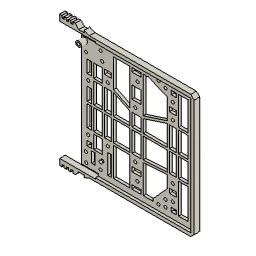
Rack and Dock v2 v74 (Autodesk Fusion 360 design; units mm, degrees)
Autodesk Fusion 360 part; units mm, degrees
(part 1 of 4)
sketch "Base Shape" plane through (0, 0, 0) normal (0, 1, 0) x (1, 0, 0) in component "Card Plate"
  line L0 (0, 0) -> (0, -50)
  line L1 (0, -50) -> (15, -50)
  line L2 (15, -50) -> (15, -53)
  line L3 (15, -53) -> (-13, -53)
  line L4 (-13, -53) -> (-13, -56.5)
  line L5 (0, 0) -> (103, 0) construction
  line L6 (103, 0) -> (103, -55)
  line L7 (103, -55) -> (15, -55)
  line L8 (15, -55) -> (9.5, -55)
  line L9 (9.5, -55) -> (5, -57)
  line L10 (5, -57) -> (5, -55)
  line L11 (15, -53) -> (15, -55) construction
  line L12 (9.5, -55) -> (5, -55) construction
  line L13 (0, -50) -> (0, -55) construction
  line L14 (5, -55) -> (0, -55)
  line L15 (-13, -56.5) -> (-3, -56.5)
  line L16 (-3, -56.5) -> (0, -55)
  line L17 (15, -52) -> (100, -52)
  line L18 (100, -52) -> (100, 0)
  line L19 (67.9969, -52) -> (67.9969, -55) construction
  line L20 (100, -22.1513) -> (103, -22.1513) construction
  line L21 (0, 0) -> (0, 50)
  line L22 (0, 50) -> (15, 50)
  line L23 (15, 50) -> (15, 53)
  line L24 (15, 53) -> (-13, 53)
  line L25 (-13, 53) -> (-13, 56.5)
  line L26 (-13, 56.5) -> (-3, 56.5)
  line L27 (-3, 56.5) -> (0, 55)
  line L28 (5, 55) -> (0, 55)
  line L29 (5, 57) -> (5, 55)
  line L30 (9.5, 55) -> (5, 57)
  line L31 (15, 55) -> (9.5, 55)
  line L32 (103, 55) -> (15, 55)
  line L33 (15, 52) -> (100, 52)
  line L34 (100, 52) -> (100, 0)
  line L35 (103, 0) -> (103, 55)
  dimension "d1" = 50
  dimension "d2" = 15
  dimension "d3" = 3
  dimension "d4" = 28
  dimension "d5" = 3.5
  dimension "d6" = 103
  dimension "d7" = 55
  dimension "d8" = 5.5
  dimension "d9" = 10
  dimension "d10" = 2
  dimension "d12" = 10
  dimension "d13" = 3
  constraint coincident L0.start L5.start
  constraint vertical L0
  constraint perpendicular L0 L1
  constraint perpendicular L1 L2
  constraint perpendicular L2 L3
  constraint perpendicular L3 L4
  constraint perpendicular L0 L5
  constraint perpendicular L5 L6
  constraint perpendicular L2 L7
  constraint parallel L7 L8
  constraint perpendicular L8 L10
  constraint vertical L11
  constraint horizontal L12
  constraint vertical L13
  constraint perpendicular L13 L14
  constraint perpendicular L4 L15
  constraint coincident L2 L17.start
  constraint perpendicular L2 L17
  constraint coincident L5 L18.end
  constraint perpendicular L5 L18
  constraint coincident L17 L19.start
  constraint coincident L7 L19.end
  constraint perpendicular L7 L19
  constraint coincident L18 L20.start
  constraint coincident L6 L20.end
  constraint perpendicular L6 L20
  constraint equal L19 L20
  constraint symmetric L0.start L5 L21.start
  constraint symmetric L0.end L5 L21.end
  constraint symmetric L1.end L5 L22.end
  constraint symmetric L2.end L5 L23.end
  constraint symmetric L3.end L5 L24.end
  constraint symmetric L4.end L5 L25.end
  constraint symmetric L6.start L5 L35.start
  constraint symmetric L5 L6.end L32.start
  constraint symmetric L5 L7.end L31.start
  constraint symmetric L5 L8.end L30.start
  constraint symmetric L5 L9.end L29.start
  constraint symmetric L5 L10.end L28.start
  constraint symmetric L5 L13.end L27.end
  constraint symmetric L5 L15.end L26.end
  constraint symmetric L5 L17.start L33.start
  constraint symmetric L5 L17.end L33.end
  constraint symmetric L5 L18.end L34.end
  measures "d1" distance of L0.start L0.end
  measures "d2" distance of L0.end L1.end
  measures "d3" distance of L1.end L2.end
  measures "d4" distance of L2.end L3.end
  measures "d5" distance of L3.end L4.end
  measures "d6" distance of L0.start L5.end
  measures "d7" distance of L5.end L6.end
  measures "d8" distance of L7.end L8.end
  measures "d9" horizontal distance of L7.end L9.end
  measures "d10" distance of L9.end L10.end
  measures "d12" distance of L4.end L15.end
  measures "d13" distance of L7 L17
extrude "Extrude1" add sketch "Base Shape" along normal blind 2 makes body 1 in component "Card Plate"
extrude "Extrude2" add sketch "Base Shape" against normal blind 3 contours L2 L3 L4 L6 L7 L8 L9 L10 L14 L15 L16 L17 L18 L23 L24 L25 L26 L27 L28 L29 L30 L31 L32 L33 L34 L35 bodies 1 in component "Card Plate"
chamfer "Chamfer1" distance 3 angle 45 2 edges at (103, -0.5, 55) (103, -0.5, -55) on bodies 1 in component "Card Plate"
sketch "Knurling" plane through (0, -3, 0) normal (0, -1, 0) x (1, 0, 0) in component "Card Plate"
  line L0 (100, -55) -> (103, -52)
  line L1 (103, -52) -> (103, 52)
  line L2 (103, 52) -> (100, 55)
  line L3 (100, 55) -> (9.5, 55)
  line L4 (9.5, 55) -> (5, 57)
  line L5 (5, 57) -> (5, 55)
  line L6 (5, 55) -> (0, 55)
  line L7 (0, 55) -> (-3, 56.5)
  line L8 (-3, 56.5) -> (-13, 56.5)
  line L9 (-13, 56.5) -> (-13, 53)
  line L10 (-13, 53) -> (15, 53)
  line L11 (15, 53) -> (15, 52)
  line L12 (15, 52) -> (100, 52)
  line L13 (100, 52) -> (100, -52)
  line L14 (100, -52) -> (15, -52)
  line L15 (15, -52) -> (15, -53)
  line L16 (15, -53) -> (-13, -53)
  line L17 (-13, -53) -> (-13, -56.5)
  line L18 (-13, -56.5) -> (-3, -56.5)
  line L19 (-3, -56.5) -> (0, -55)
  line L20 (0, -55) -> (5, -55)
  line L21 (5, -55) -> (5, -57)
  line L22 (5, -57) -> (9.5, -55)
  line L23 (9.5, -55) -> (100, -55)
  line L24 (-12, 56.5) -> (-12, 55.5)
  line L25 (-12, 55.5) -> (-11, 55.5)
  line L26 (-11, 55.5) -> (-11, 56.5)
  line L27 (0, 0) -> (100, 0) construction
  line L28 (-12, -56.5) -> (-12, -55.5)
  line L29 (-12, -55.5) -> (-11, -55.5)
  line L30 (-11, -55.5) -> (-11, -56.5)
  line L31 (-10.125, 56.5) -> (-10.125, 55.5)
  line L32 (-10.125, 55.5) -> (-9.125, 55.5)
  line L33 (-9.125, 55.5) -> (-9.125, 56.5)
  line L34 (-10.125, -56.5) -> (-10.125, -55.5)
  line L35 (-10.125, -55.5) -> (-9.125, -55.5)
  line L36 (-9.125, -55.5) -> (-9.125, -56.5)
  line L37 (-8.25, 56.5) -> (-8.25, 55.5)
  line L38 (-8.25, 55.5) -> (-7.25, 55.5)
  line L39 (-7.25, 55.5) -> (-7.25, 56.5)
  line L40 (-8.25, -56.5) -> (-8.25, -55.5)
  line L41 (-8.25, -55.5) -> (-7.25, -55.5)
  line L42 (-7.25, -55.5) -> (-7.25, -56.5)
  line L43 (-6.375, 56.5) -> (-6.375, 55.5)
  line L44 (-6.375, 55.5) -> (-5.375, 55.5)
  line L45 (-5.375, 55.5) -> (-5.375, 56.5)
  line L46 (-6.375, -56.5) -> (-6.375, -55.5)
  line L47 (-6.375, -55.5) -> (-5.375, -55.5)
  line L48 (-5.375, -55.5) -> (-5.375, -56.5)
  line L49 (-4.5, 56.5) -> (-4.5, 55.5)
  line L50 (-4.5, 55.5) -> (-3.5, 55.5)
  line L51 (-3.5, 55.5) -> (-3.5, 56.5)
  line L52 (-4.5, -56.5) -> (-4.5, -55.5)
  line L53 (-4.5, -55.5) -> (-3.5, -55.5)
  line L54 (-3.5, -55.5) -> (-3.5, -56.5)
  dimension "d19" = 1
  dimension "d20" = 1
  dimension "d21" = 1
  dimension "d24" = 7.5
  dimension "d25" = 0
  constraint coincident L8 L24.start
  constraint perpendicular L8 L24
  constraint perpendicular L24 L25
  constraint coincident L8 L26.end
  constraint perpendicular L8 L26
  constraint coincident L27.start origin
  constraint midpoint L13 L27.end
  constraint symmetric L24.start L27 L28.start
  constraint symmetric L24.end L27 L28.end
  constraint symmetric L25.end L27 L29.end
  constraint symmetric L26.end L27 L30.end
  measures "d19" distance of L24.start L24.end
  measures "d20" distance of L24.end L25.end
  measures "d21" distance of L8.end L24.start
extrude "Extrude6" cut sketch "Knurling" against normal blind 20 contours L18 L52 L53 L54 | L18 L46 L47 L48 | L8 L49 L50 L51 | L18 L40 L41 L42 | L8 L43 L44 L45 | L18 L34 L35 L36 | L8 L37 L38 L39 | L18 L28 L29 L30 | L8 L31 L32 L33 | L8 L24 L25 L26 bodies 1 in component "Card Plate"
sketch "Base Shape (2)" plane through (0, 2, 0) normal (0, 1, 0) x (-1, 0, 0) in component "Bay Body"
  line L0 (-15, -53) -> (-15, -50)
  line L1 (-15, -50) -> (0, -50)
  line L2 (0, -50) -> (0, 50)
  line L3 (0, 50) -> (-15, 50)
  line L4 (-15, 50) -> (-15, 53)
  line L5 (-5, 55) -> (0, 55)
  line L6 (-5, 57) -> (-5, 55)
  line L7 (-9.5, 55) -> (-5, 57)
  line L8 (-100, 55) -> (-9.5, 55)
  line L9 (-100, 55) -> (-103, 52)
  line L10 (-103, 52) -> (-103, 0) construction
  line L11 (-103.2, 52.0828) -> (-103.2, 0)
  line L12 (-100.0828, 55.2) -> (-103.2, 52.0828)
  line L13 (-100.0828, 55.2) -> (-9.5424, 55.2)
  line L14 (-9.5424, 55.2) -> (-4.8, 57.3078)
  line L15 (-4.8, 57.3078) -> (-4.8, 55.2)
  line L16 (-4.8, 55.2) -> (0, 55.2)
  line L17 (-103, 0) -> (0, 0) construction
  circle A0 centre (-14, 60.2) radius 2.25
  line L18 (-51.5, 0) -> (-51.5, 68.1067) construction
  circle A1 centre (-96.5, 60.2) radius 2.25
  line L19 (-96.5, 60.2) -> (-51.5, 60.2) construction
  line L20 (-14, 60.2) -> (-51.5, 60.2) construction
  line L21 (-96.5, 60.2) -> (-96.5, 55.2) construction
  line L22 (-14, 60.2) -> (-14, 55.2) construction
  line L23 (0, 55.2) -> (0, 65.2) construction
  line L24 (-108.2, 60.2) -> (-108.2, 0)
  line L25 (0, 60.2) -> (-7.3, 60.2)
  line L26 (-7.3, 60.2) -> (-7.3, 65.2)
  line L27 (-7.3, 65.2) -> (-20.7, 65.2)
  line L28 (-14, 60.2) -> (-14, 65.2) construction
  line L29 (-20.7, 60.2) -> (-51.5, 60.2)
  line L30 (-20.7, 65.2) -> (-20.7, 60.2)
  line L31 (0, 60.2) -> (0, 55.2)
  line L32 (-96.5, 60.2) -> (-96.5, 65.2) construction
  line L33 (-89.8, 65.2) -> (-103.2, 65.2)
  line L34 (-89.8, 65.2) -> (-89.8, 60.2)
  line L35 (-103.2, 65.2) -> (-103.2, 60.2)
  line L36 (-89.8, 60.2) -> (-51.5, 60.2)
  line L37 (-103.2, 60.2) -> (-108.2, 60.2)
  line L38 (-4.8, -55.2) -> (0, -55.2)
  line L39 (-4.8, -57.3078) -> (-4.8, -55.2)
  line L40 (-9.5424, -55.2) -> (-4.8, -57.3078)
  line L41 (-100.0828, -55.2) -> (-9.5424, -55.2)
  line L42 (-100.0828, -55.2) -> (-103.2, -52.0828)
  line L43 (-103.2, -52.0828) -> (-103.2, 0)
  line L44 (0, -60.2) -> (0, -55.2)
  line L45 (0, -60.2) -> (-7.3, -60.2)
  line L46 (-7.3, -60.2) -> (-7.3, -65.2)
  line L47 (-7.3, -65.2) -> (-20.7, -65.2)
  line L48 (-20.7, -65.2) -> (-20.7, -60.2)
  circle A2 centre (-14, -60.2) radius 2.25
  line L49 (-20.7, -60.2) -> (-51.5, -60.2)
  line L50 (-89.8, -60.2) -> (-51.5, -60.2)
  line L51 (-89.8, -65.2) -> (-89.8, -60.2)
  line L52 (-89.8, -65.2) -> (-103.2, -65.2)
  line L53 (-103.2, -65.2) -> (-103.2, -60.2)
  line L54 (-103.2, -60.2) -> (-108.2, -60.2)
  line L55 (-108.2, -60.2) -> (-108.2, 0)
  circle A3 centre (-96.5, -60.2) radius 2.25
  line L56 (-67.2166, 55.2) -> (-67.2166, 60.2) construction
  line L57 (-103.2, 0) -> (-108.2, 0) construction
  line L58 (8.25, -55.5) -> (8.25, -56.5)
  line L59 (8.25, -56.5) -> (9.125, -56.5)
  line L60 (9.125, -56.5) -> (9.125, -55.5)
  line L61 (9.125, -55.5) -> (10.125, -55.5)
  line L62 (10.125, -55.5) -> (10.125, -56.5)
  line L63 (10.125, -56.5) -> (11, -56.5)
  line L64 (11, -56.5) -> (11, -55.5)
  line L65 (11, -55.5) -> (12, -55.5)
  line L66 (12, -55.5) -> (12, -56.5)
  line L67 (12, -56.5) -> (13, -56.5)
  line L68 (13, -56.5) -> (13, -53)
  line L69 (13, -53) -> (-15, -53)
  line L70 (-15, 53) -> (13, 53)
  line L71 (13, 53) -> (13, 56.5)
  line L72 (13, 56.5) -> (12, 56.5)
  line L73 (12, 56.5) -> (12, 55.5)
  line L74 (12, 55.5) -> (11, 55.5)
  line L75 (11, 55.5) -> (11, 56.5)
  line L76 (11, 56.5) -> (10.125, 56.5)
  line L77 (10.125, 56.5) -> (10.125, 55.5)
  line L78 (10.125, 55.5) -> (9.125, 55.5)
  line L79 (9.125, 55.5) -> (9.125, 56.5)
  line L80 (9.125, 56.5) -> (8.25, 56.5)
  line L81 (8.25, 56.5) -> (8.25, 55.5)
  line L82 (8.25, 55.5) -> (7.25, 55.5)
  line L83 (7.25, 55.5) -> (7.25, 56.5)
  line L84 (7.25, 56.5) -> (6.375, 56.5)
  line L85 (6.375, 56.5) -> (6.375, 55.5)
  line L86 (6.375, 55.5) -> (5.375, 55.5)
  line L87 (5.375, 55.5) -> (5.375, 56.5)
  line L88 (5.375, 56.5) -> (4.5, 56.5)
  line L89 (4.5, 56.5) -> (4.5, 55.5)
  line L90 (4.5, 55.5) -> (3.5, 55.5)
  line L91 (3.5, 55.5) -> (3.5, 56.5)
  line L92 (3.5, 56.5) -> (3, 56.5)
  line L93 (3, 56.5) -> (0, 55)
  line L94 (0, 55) -> (-5, 55)
  line L95 (-5, 55) -> (-5, 57)
  line L96 (-5, 57) -> (-9.5, 55)
  line L97 (-9.5, 55) -> (-100, 55)
  line L98 (-100, 55) -> (-103, 52)
  line L99 (-103, -52) -> (-100, -55)
  line L100 (-100, -55) -> (-9.5, -55)
  line L101 (-9.5, -55) -> (-5, -57)
  line L102 (-5, -57) -> (-5, -55)
  line L103 (-5, -55) -> (0, -55)
  line L104 (0, -55) -> (3, -56.5)
  line L105 (3, -56.5) -> (3.5, -56.5)
  line L106 (3.5, -56.5) -> (3.5, -55.5)
  line L107 (3.5, -55.5) -> (4.5, -55.5)
  line L108 (4.5, -55.5) -> (4.5, -56.5)
  line L109 (4.5, -56.5) -> (5.375, -56.5)
  line L110 (5.375, -56.5) -> (5.375, -55.5)
  line L111 (5.375, -55.5) -> (6.375, -55.5)
  line L112 (6.375, -55.5) -> (6.375, -56.5)
  line L113 (6.375, -56.5) -> (7.25, -56.5)
  line L114 (7.25, -56.5) -> (7.25, -55.5)
  line L115 (7.25, -55.5) -> (8.25, -55.5)
  dimension "d28" = 0.2
  dimension "d29" = 4.5
  dimension "d30" = 4.5
  dimension "d31" = 5
  dimension "d32" = 37.5
  dimension "d33" = 5
  dimension "d35" = 13.4
  dimension "d36" = 45
  constraint coincident L9.end L10.start
  constraint coincident L17.end origin
  constraint perpendicular L2 L17
  constraint midpoint L17 L18.start
  constraint perpendicular L17 L18
  constraint coincident A1.centre L19.start
  constraint coincident L18 L19.end
  constraint perpendicular L18 L19
  constraint coincident A0.centre L20.start
  constraint perpendicular L18 L20
  constraint coincident L13 L21.end
  constraint perpendicular L13 L21
  constraint coincident L13 L22.end
  constraint perpendicular L13 L22
  constraint equal L21 L22
  constraint perpendicular L16 L23
  constraint vertical L10
  constraint perpendicular L17 L24
  constraint coincident L23 L25.start
  constraint perpendicular L23 L25
  constraint midpoint L27 L28.end
  constraint vertical L28
  constraint equal L22 L28
  constraint perpendicular L18 L29
  constraint vertical L26
  constraint perpendicular L27 L30
  constraint vertical L30
  constraint equal L26 L30
  constraint perpendicular L19 L32
  constraint equal L28 L32
  constraint perpendicular L32 L33
  constraint midpoint L32.end L33
  constraint coincident L19 L34.end
  constraint perpendicular L19 L34
  constraint perpendicular L33 L35
  constraint coincident L24 L37.end
  constraint perpendicular L24 L37
  constraint equal L27 L33
  constraint symmetric L11.start L17 L42.end
  constraint symmetric L11.end L17 L43.end
  constraint symmetric L12.start L17 L41.start
  constraint symmetric L13.end L17 L40.start
  constraint symmetric L14.end L17 L39.start
  constraint symmetric L15.end L17 L38.start
  constraint symmetric L16.end L17 L38.end
  constraint symmetric L17 A0 A2
  constraint symmetric L17 A1 A3
  constraint symmetric L17 L24.end L55.end
  constraint symmetric L17 L25.start L44.start
  constraint symmetric L17 L25.end L45.end
  constraint symmetric L17 L26.end L46.end
  constraint symmetric L17 L27.end L47.end
  constraint symmetric L17 L29.start L48.end
  constraint symmetric L17 L19.end L49.end
  constraint symmetric L17 L33.start L51.start
  constraint symmetric L17 L33.end L52.end
  constraint symmetric L17 L34.end L50.start
  constraint symmetric L17 L35.end L53.end
  constraint symmetric L17 L24.start L54.end
  constraint coincident L13 L56.start
  constraint coincident L36 L56.end
  constraint perpendicular L36 L56
  constraint perpendicular L43 L57
  constraint equal L56 L57
  constraint equal L34 L35
  measures "d29" diameter of A0
  measures "d30" diameter of A1
  measures "d31" distance of A0.centre L22.end
  measures "d32" distance of A0.centre L19.end
  measures "d33" vertical distance of L25.end L26.end
  measures "d35" distance of L26.end L27.end
  measures "d36" distance of L18 A1.centre
extrude "Extrude1'" add sketch "Base Shape (2)" against normal blind 5.5 separate body makes body 2 in component "Bay Body"
sketch "Backing Tab" plane through (0, 2, 0) normal (0, 1, 0) x (-1, 0, 0) in component "Bay Body"
  circle A0 centre (-96.5, -60.2) radius 2.25
  circle A1 centre (-96.5, 60.2) radius 2.25
  circle A2 centre (-14, -60.2) radius 2.25
  circle A3 centre (-14, 60.2) radius 2.25
  line L0 (-89.8, -65.2) -> (-89.8, -60.2)
  line L1 (-89.8, -60.2) -> (-20.7, -60.2)
  line L2 (-20.7, -60.2) -> (-20.7, -65.2)
  line L3 (-20.7, -65.2) -> (-7.3, -65.2)
  line L4 (-7.3, -65.2) -> (-7.3, -60.2)
  line L5 (-7.3, -60.2) -> (0, -60.2)
  line L6 (0, -60.2) -> (0, -55.2)
  line L7 (0, -55.2) -> (-4.8, -55.2)
  line L8 (-4.8, -55.2) -> (-4.8, -57.3078)
  line L9 (-4.8, -57.3078) -> (-9.5424, -55.2)
  line L10 (-9.5424, -55.2) -> (-100.0828, -55.2)
  line L11 (-100.0828, -55.2) -> (-103.2, -52.0828)
  line L12 (-103.2, -52.0828) -> (-103.2, 52.0828)
  line L13 (-103.2, 52.0828) -> (-100.0828, 55.2)
  line L14 (-100.0828, 55.2) -> (-9.5424, 55.2)
  line L15 (-9.5424, 55.2) -> (-4.8, 57.3078)
  line L16 (-4.8, 57.3078) -> (-4.8, 55.2)
  line L17 (-4.8, 55.2) -> (0, 55.2)
  line L18 (0, 55.2) -> (0, 60.2)
  line L19 (0, 60.2) -> (-7.3, 60.2)
  line L20 (-7.3, 60.2) -> (-7.3, 65.2)
  line L21 (-7.3, 65.2) -> (-20.7, 65.2)
  line L22 (-20.7, 65.2) -> (-20.7, 60.2)
  line L23 (-20.7, 60.2) -> (-89.8, 60.2)
  line L24 (-89.8, 60.2) -> (-89.8, 65.2)
  line L25 (-89.8, 65.2) -> (-103.2, 65.2)
  line L26 (-103.2, 65.2) -> (-103.2, 60.2)
  line L27 (-103.2, 60.2) -> (-108.2, 60.2)
  line L28 (-108.2, 60.2) -> (-108.2, -60.2)
  line L29 (-108.2, -60.2) -> (-103.2, -60.2)
  line L30 (-103.2, -60.2) -> (-103.2, -65.2)
  line L31 (-103.2, -65.2) -> (-89.8, -65.2)
  line L32 (0, 55.2) -> (0, 52)
  line L33 (0, 52) -> (-100, 52)
  line L34 (0, 0) -> (-118.983, 0) construction
  line L35 (-100, 52) -> (-100, 0)
  line L36 (0, -55.2) -> (0, -52)
  line L37 (0, -52) -> (-100, -52)
  line L38 (-100, -52) -> (-100, 0)
  dimension "d48" = 3.2
  dimension "d49" = 3.2
  constraint coincident L17.end L18.start
  constraint perpendicular L17 L32
  constraint perpendicular L32 L33
  constraint coincident L34.start origin
  constraint perpendicular L28 L34
  constraint coincident L34 L35.end
  constraint perpendicular L34 L35
  constraint symmetric L17.end L34 L6.end
  constraint symmetric L32.end L34 L36.end
  constraint symmetric L33.end L34 L37.end
  constraint symmetric L34 L35.end L38.end
  measures "d48" distance of L17.end L32.end
  measures "d49" distance of L12 L33.end
extrude "Extrude3" add sketch "Backing Tab" along normal blind 2 bodies 2 in component "Bay Body"
chamfer "Chamfer8" distance 2.5 angle 45 8 edges at (7.3, 0.25, 65.2) (20.7, 0.25, 65.2) (89.8, 0.25, 65.2) (103.2, 0.25, 65.2) (103.2, 0.25, -65.2) (89.8, 0.25, -65.2) (20.7, 0.25, -65.2) (7.3, 0.25, -65.2) on bodies 2 in component "Bay Body"
chamfer "Chamfer9" distance 2.5 angle 45 8 edges at (103.2, 0.25, 60.2) (89.8, 0.25, 60.2) (7.3, 0.25, 60.2) (20.7, 0.25, 60.2) (103.2, 0.25, -60.2) (89.8, 0.25, -60.2) (7.3, 0.25, -60.2) (20.7, 0.25, -60.2) on bodies 2 in component "Bay Body"
chamfer "Chamfer10" distance 2.5 angle 45 2 edges at (108.2, 0.25, 60.2) (108.2, 0.25, -60.2) on bodies 2 in component "Bay Body"
chamfer "Chamfer11" distance 1 angle 45 2 edges at (0, 0.25, 60.2) (0, 0.25, -60.2) on bodies 2 in component "Bay Body"
sketch "extra material near tab" plane through (0, -3.5, 0) normal (0, -1, 0) x (1, 0, 0) in component "Bay Body"
  line L0 (0, -59.2) -> (1, -60.2)
  line L1 (1, -60.2) -> (4.8, -60.2)
  line L2 (4.8, -60.2) -> (9.8, -65.2)
  line L3 (9.8, -65.2) -> (18.2, -65.2)
  line L4 (18.2, -65.2) -> (23.2, -60.2)
  line L5 (23.2, -60.2) -> (87.3, -60.2)
  line L6 (87.3, -60.2) -> (92.3, -65.2)
  line L7 (92.3, -65.2) -> (100.7, -65.2)
  line L8 (100.7, -65.2) -> (108.2, -57.7)
  line L9 (108.2, -57.7) -> (108.2, 57.7)
  line L10 (108.2, 57.7) -> (100.7, 65.2)
  line L11 (100.7, 65.2) -> (92.3, 65.2)
  line L12 (92.3, 65.2) -> (87.3, 60.2)
  line L13 (87.3, 60.2) -> (23.2, 60.2)
  line L14 (23.2, 60.2) -> (18.2, 65.2)
  line L15 (18.2, 65.2) -> (9.8, 65.2)
  line L16 (9.8, 65.2) -> (4.8, 60.2)
  line L17 (4.8, 60.2) -> (1, 60.2)
  line L18 (1, 60.2) -> (0, 59.2)
  line L19 (0, 59.2) -> (0, 55.2)
  line L20 (0, 55.2) -> (4.8, 55.2)
  line L21 (4.8, 55.2) -> (4.8, 57.3078)
  line L22 (4.8, 57.3078) -> (9.5424, 55.2)
  line L23 (9.5424, 55.2) -> (100.0828, 55.2)
  line L24 (100.0828, 55.2) -> (103.2, 52.0828)
  line L25 (103.2, 52.0828) -> (103.2, -52.0828)
  line L26 (103.2, -52.0828) -> (100.0828, -55.2)
  line L27 (100.0828, -55.2) -> (9.5424, -55.2)
  line L28 (9.5424, -55.2) -> (4.8, -57.3078)
  line L29 (4.8, -57.3078) -> (4.8, -55.2)
  line L30 (4.8, -55.2) -> (0, -55.2)
  line L31 (0, -55.2) -> (0, -59.2)
  circle A0 centre (96.5, -60.2) radius 2.25
  circle A1 centre (96.5, 60.2) radius 2.25
  circle A2 centre (14, -60.2) radius 2.25
  circle A3 centre (14, 60.2) radius 2.25
  line L32 (0, 59.2) -> (2.1078, 61.3078)
  line L33 (2.1078, 61.3078) -> (5.9078, 61.3078)
  line L34 (0, 0) -> (31.4782, 0) construction
  line L35 (0, -59.2) -> (2.1078, -61.3078)
  line L36 (2.1078, -61.3078) -> (5.9078, -61.3078)
  dimension "d56" = 4
  constraint coincident L18.end L19.start
  constraint parallel L18 L32
  constraint coincident L16 L33.end
  constraint parallel L17 L33
  constraint coincident L34.start origin
  constraint perpendicular L25 L34
  constraint symmetric L18.end L34 L0.start
  constraint symmetric L32.end L34 L35.end
  constraint symmetric L33.end L34 L36.end
  measures "d56" distance of L21.end L33
extrude "Extrude4" add sketch "extra material near tab" against normal blind 7.5 contours L1 L2 L35 L36 | L16 L17 L32 L33 bodies 2 in component "Bay Body"
sketch "Base Shape (3)" plane through (0, 4, 0) normal (0, 1, 0) x (-1, 0, 0) in component "End Frame A"
  circle A0 centre (-14, 60.2) radius 2.25
  circle A1 centre (-14, -60.2) radius 2.25
  circle A2 centre (-96.5, 60.2) radius 2.25
  circle A3 centre (-96.5, -60.2) radius 2.25
  line L0 (-2.1078, -61.3078) -> (0, -59.2)
  line L1 (0, -59.2) -> (0, -52)
  line L2 (0, -52) -> (-100, -52)
  line L3 (-100, -52) -> (-100, 52)
  line L4 (-100, 52) -> (0, 52)
  line L5 (0, 52) -> (0, 59.2)
  line L6 (0, 59.2) -> (-2.1078, 61.3078)
  line L7 (-2.1078, 61.3078) -> (-5.9078, 61.3078)
  line L8 (-5.9078, 61.3078) -> (-9.8, 65.2)
  line L9 (-9.8, 65.2) -> (-18.2, 65.2)
  line L10 (-18.2, 65.2) -> (-23.2, 60.2)
  line L11 (-23.2, 60.2) -> (-87.3, 60.2)
  line L12 (-87.3, 60.2) -> (-92.3, 65.2)
  line L13 (-92.3, 65.2) -> (-100.7, 65.2)
  line L14 (-100.7, 65.2) -> (-108.2, 57.7)
  line L15 (-108.2, 57.7) -> (-108.2, -57.7)
  line L16 (-108.2, -57.7) -> (-100.7, -65.2)
  line L17 (-100.7, -65.2) -> (-92.3, -65.2)
  line L18 (-92.3, -65.2) -> (-87.3, -60.2)
  line L19 (-87.3, -60.2) -> (-23.2, -60.2)
  line L20 (-23.2, -60.2) -> (-18.2, -65.2)
  line L21 (-18.2, -65.2) -> (-9.8, -65.2)
  line L22 (-9.8, -65.2) -> (-5.9078, -61.3078)
  line L23 (-5.9078, -61.3078) -> (-2.1078, -61.3078)
  line L24 (-96.5, 60.2) -> (-14, 60.2) construction
  line L25 (-96.5, -60.2) -> (-14, -60.2) construction
  line L26 (-55.25, -60.2) -> (-55.25, 60.2) construction
  line L27 (-55.25, 0) -> (-108.2, 0) construction
  line L28 (-55.25, 60.2) -> (-87.3, 60.2)
  line L29 (-87.3, 60.2) -> (-92.3, 65.2)
  line L30 (-92.3, 65.2) -> (-100.7, 65.2)
  line L31 (-100.7, 65.2) -> (-108.2, 57.7)
  line L32 (-108.2, 57.7) -> (-108.2, 0)
  circle A4 centre (-96.5, 60.2) radius 2.25
  line L33 (-55.25, 60.2) -> (-23.2, 60.2)
  line L34 (-23.2, 60.2) -> (-18.2, 65.2)
  line L35 (-18.2, 65.2) -> (-9.8, 65.2)
  line L36 (-9.8, 65.2) -> (-2.3, 57.7)
  line L37 (-2.3, 57.7) -> (-2.3, 0)
  circle A5 centre (-14, 60.2) radius 2.25
  line L38 (-108.2, -57.7) -> (-108.2, 0)
  line L39 (-100.7, -65.2) -> (-108.2, -57.7)
  line L40 (-92.3, -65.2) -> (-100.7, -65.2)
  line L41 (-87.3, -60.2) -> (-92.3, -65.2)
  line L42 (-55.25, -60.2) -> (-87.3, -60.2)
  line L43 (-23.2, -60.2) -> (-18.2, -65.2)
  line L44 (-55.25, -60.2) -> (-23.2, -60.2)
  line L45 (-18.2, -65.2) -> (-9.8, -65.2)
  line L46 (-9.8, -65.2) -> (-2.3, -57.7)
  line L47 (-2.3, -57.7) -> (-2.3, 0)
  circle A6 centre (-96.5, -60.2) radius 2.25
  circle A7 centre (-14, -60.2) radius 2.25
  constraint coincident A2.centre L24.start
  constraint coincident A0.centre L24.end
  constraint coincident A3.centre L25.start
  constraint coincident A1.centre L25.end
  constraint midpoint L25 L26.start
  constraint midpoint L24 L26.end
  constraint midpoint L26 L27.start
  constraint midpoint L15 L27.end
  constraint coincident L11.end L12.start
  constraint coincident L12.end L13.start
  constraint coincident L13.end L14.start
  constraint coincident L14.end L15.start
  constraint concentric A2 A4
  constraint symmetric L28.start L26 L33.start
  constraint symmetric L26 L27.end L37.end
  constraint symmetric L26 L11.end L10.end
  constraint symmetric L26 L12.end L9.end
  constraint symmetric L26 L13.end L8.end
  constraint symmetric L26 L14.end L36.end
  constraint symmetric L26 A4 A5
  constraint symmetric L26.end L27 L26.start
  constraint symmetric L32.end L27 L38.end
  constraint symmetric L27 L11.end L18.end
  constraint symmetric L27 L12.end L17.end
  constraint symmetric L27 L13.end L16.end
  constraint symmetric L27 L14.end L15.end
  constraint symmetric L27 A4 A6
  constraint symmetric L27 L26.end L26.start
  constraint symmetric L27 L10.end L19.end
  constraint symmetric L27 L9.end L20.end
  constraint symmetric L27 L8.end L21.end
  constraint symmetric L27 L36.end L46.end
  constraint symmetric L27 L37.end L47.end
  constraint symmetric L27 A5 A7
extrude "Extrude1''" add sketch "Base Shape (3)" along normal blind 3 separate body contours A0 A5 | A1 A7 | A2 A4 | A3 A6 | L2 L3 L4 L8 L9 L10 L11 L12 L13 L14 L15 L16 L17 L18 L19 L20 L21 L22 L28 L29 L30 L31 L32 L33 L34 L35 L36 L37 L38 L39 L40 L41 L42 L43 L44 L45 L46 L47 | L2 L3 L4 L37 L47 makes body 3 in component "End Frame A"
sketch "Bar Holder" plane through (0, 4, 0) normal (0, -1, 0) x (1, 0, 0) in component "End Frame A"
  line L0 (23.2, -60.2) -> (87.3, -60.2)
  line L1 (87.3, -60.2) -> (92.3, -65.2)
  line L2 (92.3, -65.2) -> (100.7, -65.2)
  line L3 (100.7, -65.2) -> (108.2, -57.7)
  line L4 (108.2, -57.7) -> (108.2, 57.7)
  line L5 (108.2, 57.7) -> (100.7, 65.2)
  line L6 (100.7, 65.2) -> (92.3, 65.2)
  line L7 (92.3, 65.2) -> (87.3, 60.2)
  line L8 (87.3, 60.2) -> (23.2, 60.2)
  line L9 (23.2, 60.2) -> (18.2, 65.2)
  line L10 (18.2, 65.2) -> (9.8, 65.2)
  line L11 (9.8, 65.2) -> (2.3, 57.7)
  line L12 (2.3, 57.7) -> (2.3, -57.7)
  line L13 (2.3, -57.7) -> (9.8, -65.2)
  line L14 (9.8, -65.2) -> (18.2, -65.2)
  line L15 (18.2, -65.2) -> (23.2, -60.2)
  circle A0 centre (14, 60.2) radius 2.25
  line L16 (55.25, 60.2) -> (55.25, -60.2) construction
  line L17 (108.2, 0) -> (2.3, 0) construction
  line L18 (11.75, 60.2) -> (16.25, 60.2) construction
  line L19 (16.25, 60.2) -> (16.25, 65.2)
  line L20 (16.25, 65.2) -> (19.7855, 68.7355)
  line L21 (11.75, 65.2) -> (16.75, 65.2) construction
  line L22 (19.7855, 68.7355) -> (22.5433, 68.7355)
  line L23 (22.5433, 68.7355) -> (18.6039, 64.7961)
  line L24 (22.5433, 68.7355) -> (26.8209, 68.7355) construction
  line L25 (18.2, 65.2) -> (18.2, 60.2)
  circle A1 centre (14, 60.2) radius 4.2
  line L26 (18.4731, 67.4231) -> (19.852, 66.0443) construction
  line L27 (18.6039, 64.7961) -> (18.2, 64.3923)
  line L28 (14, 60.2) -> (14, 62.45) construction
  line L29 (5.4567, 68.7355) -> (9.3961, 64.7961)
  line L30 (8.2145, 68.7355) -> (5.4567, 68.7355)
  line L31 (11.75, 65.2) -> (8.2145, 68.7355)
  line L32 (11.75, 60.2) -> (11.75, 65.2)
  line L33 (9.8, 65.2) -> (9.8, 60.2)
  line L34 (9.3961, 64.7961) -> (9.8, 64.3923)
  circle A2 centre (14, 60.2) radius 2.25
  circle A3 centre (96.5, 60.2) radius 2.25
  circle A4 centre (14, -60.2) radius 2.25
  line L35 (98.75, 65.2) -> (102.2855, 68.7355)
  line L36 (102.2855, 68.7355) -> (105.0433, 68.7355)
  line L37 (105.0433, 68.7355) -> (101.1039, 64.7961)
  line L38 (101.1039, 64.7961) -> (100.7, 64.3923)
  line L39 (100.7, 65.2) -> (100.7, 60.2)
  line L40 (98.75, 60.2) -> (98.75, 65.2)
  circle A5 centre (96.5, 60.2) radius 4.2
  circle A6 centre (96.5, 60.2) radius 2.25
  line L41 (94.25, 60.2) -> (94.25, 65.2)
  line L42 (92.3, 65.2) -> (92.3, 60.2)
  line L43 (91.8961, 64.7961) -> (92.3, 64.3923)
  line L44 (87.9567, 68.7355) -> (91.8961, 64.7961)
  line L45 (94.25, 65.2) -> (90.7145, 68.7355)
  line L46 (90.7145, 68.7355) -> (87.9567, 68.7355)
  line L47 (16.25, -55.2) -> (19.7855, -51.6645)
  line L48 (19.7855, -51.6645) -> (22.5433, -51.6645)
  line L49 (22.5433, -51.6645) -> (18.6039, -55.6039)
  line L50 (18.6039, -55.6039) -> (18.2, -56.0077)
  line L51 (18.2, -55.2) -> (18.2, -60.2)
  line L52 (16.25, -60.2) -> (16.25, -55.2)
  circle A7 centre (14, -60.2) radius 4.2
  circle A8 centre (14, -60.2) radius 2.25
  line L53 (11.75, -60.2) -> (11.75, -55.2)
  line L54 (9.8, -55.2) -> (9.8, -60.2)
  line L55 (9.3961, -55.6039) -> (9.8, -56.0077)
  line L56 (5.4567, -51.6645) -> (9.3961, -55.6039)
  line L57 (11.75, -55.2) -> (8.2145, -51.6645)
  line L58 (8.2145, -51.6645) -> (5.4567, -51.6645)
  line L59 (98.75, -55.2) -> (102.2855, -51.6645)
  line L60 (102.2855, -51.6645) -> (105.0433, -51.6645)
  line L61 (105.0433, -51.6645) -> (101.1039, -55.6039)
  line L62 (101.1039, -55.6039) -> (100.7, -56.0077)
  line L63 (100.7, -55.2) -> (100.7, -60.2)
  line L64 (98.75, -60.2) -> (98.75, -55.2)
  circle A9 centre (96.5, -60.2) radius 4.2
  circle A10 centre (96.5, -60.2) radius 2.25
  line L65 (94.25, -60.2) -> (94.25, -55.2)
  line L66 (92.3, -55.2) -> (92.3, -60.2)
  line L67 (91.8961, -55.6039) -> (92.3, -56.0077)
  line L68 (87.9567, -51.6645) -> (91.8961, -55.6039)
  line L69 (94.25, -55.2) -> (90.7145, -51.6645)
  line L70 (90.7145, -51.6645) -> (87.9567, -51.6645)
  dimension "d70" = 5
  dimension "d71" = 5
  dimension "d72" = 5
  dimension "d76" = 135
  dimension "d77" = 1.95
  dimension "d78" = 1.95
  dimension "d79" = 82.5
  dimension "d80" = 120.4
  dimension "d83" = 82.5
  dimension "d84" = -120.4
  constraint midpoint L8 L16.start
  constraint midpoint L0 L16.end
  constraint midpoint L4 L17.start
  constraint midpoint L12 L17.end
  constraint coincident A0 L18.start
  constraint coincident A0 L18.end
  constraint perpendicular L12 L18
  constraint perpendicular L18 L19
  constraint perpendicular L9 L20
  constraint horizontal L21
  constraint horizontal L22
  constraint horizontal L24
  constraint coincident L9 L23.end
  constraint coincident L9.end L10.start
  constraint perpendicular L10 L25
  constraint coincident L20 L26.start
  constraint coincident L23 L26.end
  constraint perpendicular L23 L26
  constraint coincident L25 L27.end
  constraint perpendicular L9 L27
  constraint coincident A0.centre A1.centre
  constraint coincident A0 L28.end
  constraint perpendicular L18 L28
  constraint symmetric L18.end L28 L18.start
  constraint symmetric L19.end L28 L21.start
  constraint symmetric L20.end L28 L30.start
  constraint symmetric L22.end L28 L29.start
  constraint symmetric L23.end L28 L29.end
  constraint symmetric L9.end L28 L10.end
  constraint symmetric L25.end L28 L33.end
  constraint symmetric L27.end L28 L34.end
  measures "d70" distance of L18.end L19.end
  measures "d71" distance of L18.start L21.start
  measures "d72" distance of L19.end L20.end
  measures "d76" angle of L23 L24
  measures "d78" distance of L26.start L26.end
  measures "d79" distance of A0.centre A3.centre
  measures "d80" distance of A0.centre A4.centre
extrude "Extrude2'" add sketch "Bar Holder" along normal blind 5 contours L10 L11 L29 L30 L31 | L11 L33 L34 | L5 L38 L39 | L5 L6 L35 L36 L37 | L10 A1 L32 L33 | L6 L39 L40 A5 | A0 L19 A1 L32 A2 | A3 L40 A5 A6 L41 | L9 L10 L20 L22 L23 | L10 L19 L25 A1 | L6 A5 L41 L42 | L6 L7 L44 L45 L46 | L9 L25 L27 | L7 L42 L43 | A4 L52 A7 A8 L53 | L47 L48 L49 L50 L51 L52 A7 | A7 L53 L54 L55 L56 L57 L58 | L59 L60 L61 L62 L63 L64 A9 | L64 A9 A10 L65 | A9 L65 L66 L67 L68 L69 L70 picked at (17.526, 59.8796) picked at (100.0344, 59.9913) picked at (17.526, -60.5204) picked at (100.0344, -60.4087) bodies 3 in component "End Frame A"
extrude "Extrude3'" add 4 faces at (20.3109, 4, 67.4224) (7.6891, 4, 67.4224) (102.8109, 4, 67.4224) (90.1891, 4, 67.4224) along direction (0, 1, 0) blind 3 on bodies 3 bodies 3 in component "End Frame A"
sketch "Top Fill Ins" plane through (0, 7, 0) normal (0, 1, 0) x (-1, 0, 0) in component "End Frame A"
  line L0 (-87.3, -60.2) -> (-23.2, -60.2)
  line L1 (-23.2, -60.2) -> (-18.2, -65.2)
  line L2 (-18.2, -65.2) -> (-9.8, -65.2)
  line L3 (-9.8, -65.2) -> (-2.3, -57.7)
  line L4 (-2.3, -57.7) -> (-2.3, 57.7)
  line L5 (-2.3, 57.7) -> (-9.3961, 64.7961)
  line L6 (-9.3961, 64.7961) -> (-5.4567, 68.7355)
  line L7 (-5.4567, 68.7355) -> (-8.2145, 68.7355)
  line L8 (-8.2145, 68.7355) -> (-11.75, 65.2)
  line L9 (-11.75, 65.2) -> (-16.25, 65.2)
  line L10 (-16.25, 65.2) -> (-19.7855, 68.7355)
  line L11 (-19.7855, 68.7355) -> (-22.5433, 68.7355)
  line L12 (-22.5433, 68.7355) -> (-18.6039, 64.7961)
  line L13 (-18.6039, 64.7961) -> (-23.2, 60.2)
  line L14 (-23.2, 60.2) -> (-87.3, 60.2)
  line L15 (-87.3, 60.2) -> (-91.8961, 64.7961)
  line L16 (-91.8961, 64.7961) -> (-87.9567, 68.7355)
  line L17 (-87.9567, 68.7355) -> (-90.7145, 68.7355)
  line L18 (-90.7145, 68.7355) -> (-94.25, 65.2)
  line L19 (-94.25, 65.2) -> (-98.75, 65.2)
  line L20 (-98.75, 65.2) -> (-102.2855, 68.7355)
  line L21 (-102.2855, 68.7355) -> (-105.0433, 68.7355)
  line L22 (-105.0433, 68.7355) -> (-101.1039, 64.7961)
  line L23 (-101.1039, 64.7961) -> (-108.2, 57.7)
  line L24 (-108.2, 57.7) -> (-108.2, -57.7)
  line L25 (-108.2, -57.7) -> (-100.7, -65.2)
  line L26 (-100.7, -65.2) -> (-92.3, -65.2)
  line L27 (-92.3, -65.2) -> (-87.3, -60.2)
  line L28 (-5.4567, 68.7355) -> (-5.4567, 60.8567)
  line L29 (-22.5433, 68.7355) -> (-22.5433, 60.8567)
  line L30 (-87.9567, 68.7355) -> (-87.9567, 60.8567)
  line L31 (-105.0433, 68.7355) -> (-105.0433, 60.8567)
  constraint coincident L6.end L7.start
  constraint coincident L5 L28.end
  constraint perpendicular L7 L28
  constraint coincident L11.end L12.start
  constraint coincident L13 L29.end
  constraint perpendicular L11 L29
  constraint coincident L16.end L17.start
  constraint coincident L15 L30.end
  constraint perpendicular L17 L30
  constraint coincident L21.end L22.start
  constraint coincident L23 L31.end
  constraint perpendicular L21 L31
extrude "Extrude4'" add sketch "Top Fill Ins" against normal blind 3 contours L22 L23 L31 | L5 L6 L28 | L15 L16 L30 | L12 L13 L29 bodies 3 in component "End Frame A"
sketch "Rear Sockets" plane through (0, 7, 0) normal (0, 1, 0) x (-1, 0, 0) in component "End Frame A"
  line L0 (-87.3, -60.2) -> (-23.2, -60.2)
  line L1 (-23.2, -60.2) -> (-18.2, -65.2)
  line L2 (-18.2, -65.2) -> (-9.8, -65.2)
  line L3 (-9.8, -65.2) -> (-2.3, -57.7)
  line L4 (-2.3, -57.7) -> (-2.3, 57.7)
  line L5 (-2.3, 57.7) -> (-5.4567, 60.8567)
  line L6 (-5.4567, 60.8567) -> (-5.4567, 68.7355)
  line L7 (-5.4567, 68.7355) -> (-8.2145, 68.7355)
  line L8 (-8.2145, 68.7355) -> (-11.75, 65.2)
  line L9 (-11.75, 65.2) -> (-16.25, 65.2)
  line L10 (-16.25, 65.2) -> (-19.7855, 68.7355)
  line L11 (-19.7855, 68.7355) -> (-22.5433, 68.7355)
  line L12 (-22.5433, 68.7355) -> (-22.5433, 60.8567)
  line L13 (-22.5433, 60.8567) -> (-23.2, 60.2)
  line L14 (-23.2, 60.2) -> (-87.3, 60.2)
  line L15 (-87.3, 60.2) -> (-87.9567, 60.8567)
  line L16 (-87.9567, 60.8567) -> (-87.9567, 68.7355)
  line L17 (-87.9567, 68.7355) -> (-90.7145, 68.7355)
  line L18 (-90.7145, 68.7355) -> (-94.25, 65.2)
  line L19 (-94.25, 65.2) -> (-98.75, 65.2)
  line L20 (-98.75, 65.2) -> (-102.2855, 68.7355)
  line L21 (-102.2855, 68.7355) -> (-105.0433, 68.7355)
  line L22 (-105.0433, 68.7355) -> (-105.0433, 60.8567)
  line L23 (-105.0433, 60.8567) -> (-108.2, 57.7)
  line L24 (-108.2, 57.7) -> (-108.2, -57.7)
  line L25 (-108.2, -57.7) -> (-100.7, -65.2)
  line L26 (-100.7, -65.2) -> (-92.3, -65.2)
  line L27 (-92.3, -65.2) -> (-87.3, -60.2)
  circle A0 centre (-14, 60.2) radius 2.25
  circle A1 centre (-96.5, 60.2) radius 2.25
  circle A2 centre (-14, -60.2) radius 2.25
  circle A3 centre (-96.5, -60.2) radius 2.25
  circle A4 centre (-96.5, 60.2) radius 1.5
  circle A5 centre (-14, 60.2) radius 1.5
  circle A6 centre (-96.5, -60.2) radius 1.5
  circle A7 centre (-14, -60.2) radius 1.5
  dimension "d91" = 3
  dimension "d92" = 3
  dimension "d93" = 3
  dimension "d94" = 3
  constraint concentric A1 A4
  constraint concentric A0 A5
  constraint concentric A3 A6
  constraint concentric A2 A7
  measures "d91" diameter of A4
  measures "d92" diameter of A5
  measures "d93" diameter of A6
  measures "d94" diameter of A7
extrude "Extrude5" cut sketch "Rear Sockets" against normal blind 1.5 contours A4 | A5 | A6 | A7 bodies 3 in component "End Frame A"
sketch "Cut Outs" plane through (0, 4, 0) normal (0, -1, 0) x (1, 0, 0) in component "End Frame A"
  arc A0 (94.25, -60.2) -> (98.75, -60.2) centre (96.5, -60.2) ccw
  line L0 (98.75, -60.2) -> (98.75, -55.2)
  line L1 (98.75, -55.2) -> (102.2855, -51.6645)
  line L2 (102.2855, -51.6645) -> (105.0433, -51.6645)
  line L3 (105.0433, -51.6645) -> (100.7, -56.0077)
  line L4 (100.7, -56.0077) -> (100.7, -60.2)
  arc A1 (92.3, -60.2) -> (100.7, -60.2) centre (96.5, -60.2) ccw
  line L5 (92.3, -60.2) -> (92.3, -56.0077)
  line L6 (92.3, -56.0077) -> (87.9567, -51.6645)
  line L7 (87.9567, -51.6645) -> (90.7145, -51.6645)
  line L8 (90.7145, -51.6645) -> (94.25, -55.2)
  line L9 (94.25, -55.2) -> (94.25, -60.2)
  line L10 (22.5433, 68.7355) -> (18.2, 64.3923)
  line L11 (18.2, 64.3923) -> (18.2, 60.2)
  arc A2 (9.8, 60.2) -> (18.2, 60.2) centre (14, 60.2) ccw
  line L12 (9.8, 60.2) -> (9.8, 64.3923)
  line L13 (9.8, 64.3923) -> (5.4567, 68.7355)
  line L14 (5.4567, 68.7355) -> (5.4567, 60.8567)
  line L15 (5.4567, 60.8567) -> (2.3, 57.7)
  line L16 (2.3, 57.7) -> (2.3, -57.7)
  line L17 (2.3, -57.7) -> (9.8, -65.2)
  line L18 (9.8, -65.2) -> (18.2, -65.2)
  line L19 (18.2, -65.2) -> (23.2, -60.2)
  line L20 (23.2, -60.2) -> (87.3, -60.2)
  line L21 (87.3, -60.2) -> (92.3, -65.2)
  line L22 (92.3, -65.2) -> (100.7, -65.2)
  line L23 (100.7, -65.2) -> (108.2, -57.7)
  line L24 (108.2, -57.7) -> (108.2, 57.7)
  line L25 (108.2, 57.7) -> (105.0433, 60.8567)
  line L26 (105.0433, 60.8567) -> (105.0433, 68.7355)
  line L27 (105.0433, 68.7355) -> (100.7, 64.3923)
  line L28 (100.7, 64.3923) -> (100.7, 60.2)
  arc A3 (92.3, 60.2) -> (100.7, 60.2) centre (96.5, 60.2) ccw
  line L29 (92.3, 60.2) -> (92.3, 64.3923)
  line L30 (92.3, 64.3923) -> (87.9567, 68.7355)
  line L31 (87.9567, 68.7355) -> (87.9567, 60.8567)
  line L32 (87.9567, 60.8567) -> (87.3, 60.2)
  line L33 (87.3, 60.2) -> (23.2, 60.2)
  line L34 (23.2, 60.2) -> (22.5433, 60.8567)
  line L35 (22.5433, 60.8567) -> (22.5433, 68.7355)
  arc A4 (11.75, -60.2) -> (16.25, -60.2) centre (14, -60.2) ccw
  line L36 (16.25, -60.2) -> (16.25, -55.2)
  line L37 (16.25, -55.2) -> (19.7855, -51.6645)
  line L38 (19.7855, -51.6645) -> (22.5433, -51.6645)
  line L39 (22.5433, -51.6645) -> (18.2, -56.0077)
  line L40 (18.2, -56.0077) -> (18.2, -60.2)
  arc A5 (9.8, -60.2) -> (18.2, -60.2) centre (14, -60.2) ccw
  line L41 (9.8, -60.2) -> (9.8, -56.0077)
  line L42 (9.8, -56.0077) -> (5.4567, -51.6645)
  line L43 (5.4567, -51.6645) -> (8.2145, -51.6645)
  line L44 (8.2145, -51.6645) -> (11.75, -55.2)
  line L45 (11.75, -55.2) -> (11.75, -60.2)
  line L46 (2.3, 0) -> (108.2, 0) construction
  line L47 (55.25, 60.2) -> (55.25, -60.2) construction
  line L48 (96.5, 60.2) -> (14, -60.2) construction
  line L49 (14, 60.2) -> (96.5, -60.2) construction
  line L50 (9.8754, 57.3738) -> (92.3754, -63.0262)
  line L51 (18.1246, 63.0262) -> (100.6246, -57.3738)
  line L52 (92.3754, 63.0262) -> (9.8754, -57.3738)
  line L53 (100.6246, 57.3738) -> (18.1246, -63.0262)
  line L54 (12.3, 50.2) -> (98.2, 50.2)
  line L55 (98.2, 50.2) -> (98.2, -50.2)
  line L56 (98.2, -50.2) -> (12.3, -50.2)
  line L57 (12.3, -50.2) -> (12.3, 50.2)
  line L58 (65.7361, 50.2) -> (65.7361, 60.2) construction
  line L59 (98.2, 22.5023) -> (108.2, 22.5023) construction
  line L60 (70.3141, -50.2) -> (70.3141, -60.2) construction
  line L61 (12.3, 10.9227) -> (2.3, 10.9227) construction
  dimension "d97" = 5
  dimension "d98" = -5
  dimension "d99" = 5
  dimension "d100" = -5
  dimension "d101" = 10
  constraint midpoint L16 L46.start
  constraint midpoint L24 L46.end
  constraint midpoint L33 L47.start
  constraint midpoint L20 L47.end
  constraint coincident A3.centre L48.start
  constraint coincident A4.centre A5.centre
  constraint coincident A2.centre L49.start
  constraint coincident A0.centre A1.centre
  constraint horizontal L54
  constraint vertical L55
  constraint horizontal L56
  constraint vertical L57
  constraint coincident L54 L58.start
  constraint coincident L33 L58.end
  constraint perpendicular L33 L58
  constraint coincident L55 L59.start
  constraint coincident L24 L59.end
  constraint perpendicular L24 L59
  constraint coincident L56 L60.start
  constraint coincident L20 L60.end
  constraint perpendicular L20 L60
  constraint coincident L57 L61.start
  constraint coincident L16 L61.end
  constraint perpendicular L16 L61
  constraint equal L58 L61
  constraint equal L58 L59
  constraint equal L59 L60
  measures "d101" distance of L16 L57
extrude "Extrude6'" cut sketch "Cut Outs" against normal blind 15 contours L51 L52 L54 | L50 L52 L54 L56 L57 | L51 L53 L54 L55 L56 | L50 L53 L56 bodies 3 in component "End Frame A"
chamfer "Chamfer1'" distance 1 angle 45 12 edges at (5.4567, 1.5, 68.7355) (5.4567, 5.5, 68.7355) (22.5433, 1.5, 68.7355) (22.5433, 5.5, 68.7355) (87.9567, 1.5, 68.7355) (87.9567, 5.5, 68.7355) (105.0433, 1.5, 68.7355) (105.0433, 5.5, 68.7355) (5.4567, 1.5, -51.6645) (22.5433, 1.5, -51.6645) (87.9567, 1.5, -51.6645) (105.0433, 1.5, -51.6645) on bodies 3 in component "End Frame A"
sketch "Fill In After Chamfer" plane through (0, 4, 0) normal (0, -1, 0) x (1, 0, 0) in component "End Frame A"
  line L0 (105.0433, 67.7355) -> (104.0433, 68.7355)
  line L1 (104.0433, 68.7355) -> (104.3361, 68.0284)
  line L2 (104.3361, 68.0284) -> (100.7, 64.3923)
  line L3 (100.7, 64.3923) -> (100.7, 60.2)
  arc A0 (92.3, 60.2) -> (100.7, 60.2) centre (96.5, 60.2) ccw
  line L4 (92.3, 60.2) -> (92.3, 64.3923)
  line L5 (92.3, 64.3923) -> (88.6639, 68.0284)
  line L6 (88.6639, 68.0284) -> (88.9567, 68.7355)
  line L7 (88.9567, 68.7355) -> (87.9567, 67.7355)
  line L8 (87.9567, 67.7355) -> (87.9567, 60.8567)
  line L9 (87.9567, 60.8567) -> (87.3, 60.2)
  line L10 (87.3, 60.2) -> (23.2, 60.2)
  line L11 (23.2, 60.2) -> (22.5433, 60.8567)
  line L12 (22.5433, 60.8567) -> (22.5433, 67.7355)
  line L13 (22.5433, 67.7355) -> (21.5433, 68.7355)
  line L14 (21.5433, 68.7355) -> (21.8361, 68.0284)
  line L15 (21.8361, 68.0284) -> (18.2, 64.3923)
  line L16 (18.2, 64.3923) -> (18.2, 60.2)
  arc A1 (9.8, 60.2) -> (18.2, 60.2) centre (14, 60.2) ccw
  line L17 (9.8, 60.2) -> (9.8, 64.3923)
  line L18 (9.8, 64.3923) -> (6.1639, 68.0284)
  line L19 (6.1639, 68.0284) -> (6.4567, 68.7355)
  line L20 (6.4567, 68.7355) -> (5.4567, 67.7355)
  line L21 (5.4567, 67.7355) -> (5.4567, 60.8567)
  line L22 (5.4567, 60.8567) -> (2.3, 57.7)
  line L23 (2.3, 57.7) -> (2.3, -57.7)
  line L24 (2.3, -57.7) -> (9.8, -65.2)
  line L25 (9.8, -65.2) -> (18.2, -65.2)
  line L26 (18.2, -65.2) -> (23.2, -60.2)
  line L27 (23.2, -60.2) -> (87.3, -60.2)
  line L28 (87.3, -60.2) -> (92.3, -65.2)
  line L29 (92.3, -65.2) -> (100.7, -65.2)
  line L30 (100.7, -65.2) -> (108.2, -57.7)
  line L31 (108.2, -57.7) -> (108.2, 57.7)
  line L32 (108.2, 57.7) -> (105.0433, 60.8567)
  line L33 (105.0433, 60.8567) -> (105.0433, 67.7355)
  line L34 (55.25, 8.8457) -> (26.9133, 50.2)
  line L35 (26.9133, 50.2) -> (83.5867, 50.2)
  line L36 (83.5867, 50.2) -> (55.25, 8.8457)
  line L37 (95.709, -50.2) -> (61.3112, 0)
  line L38 (61.3112, 0) -> (95.709, 50.2)
  line L39 (95.709, 50.2) -> (98.2, 50.2)
  line L40 (98.2, 50.2) -> (98.2, -50.2)
  line L41 (98.2, -50.2) -> (95.709, -50.2)
  line L42 (49.1888, 0) -> (14.791, -50.2)
  line L43 (14.791, -50.2) -> (12.3, -50.2)
  line L44 (12.3, -50.2) -> (12.3, 50.2)
  line L45 (12.3, 50.2) -> (14.791, 50.2)
  line L46 (14.791, 50.2) -> (49.1888, 0)
  line L47 (83.5867, -50.2) -> (26.9133, -50.2)
  line L48 (26.9133, -50.2) -> (55.25, -8.8457)
  line L49 (55.25, -8.8457) -> (83.5867, -50.2)
  arc A2 (94.25, -60.2) -> (98.75, -60.2) centre (96.5, -60.2) ccw
  line L50 (98.75, -60.2) -> (98.75, -55.2)
  line L51 (98.75, -55.2) -> (102.2855, -51.6645)
  line L52 (102.2855, -51.6645) -> (104.0433, -51.6645)
  line L53 (104.0433, -51.6645) -> (104.3361, -52.3716)
  line L54 (104.3361, -52.3716) -> (100.7, -56.0077)
  line L55 (100.7, -56.0077) -> (100.7, -60.2)
  arc A3 (92.3, -60.2) -> (100.7, -60.2) centre (96.5, -60.2) ccw
  line L56 (92.3, -60.2) -> (92.3, -56.0077)
  line L57 (92.3, -56.0077) -> (88.6639, -52.3716)
  line L58 (88.6639, -52.3716) -> (88.9567, -51.6645)
  line L59 (88.9567, -51.6645) -> (90.7145, -51.6645)
  line L60 (90.7145, -51.6645) -> (94.25, -55.2)
  line L61 (94.25, -55.2) -> (94.25, -60.2)
  arc A4 (11.75, -60.2) -> (16.25, -60.2) centre (14, -60.2) ccw
  line L62 (16.25, -60.2) -> (16.25, -55.2)
  line L63 (16.25, -55.2) -> (19.7855, -51.6645)
  line L64 (19.7855, -51.6645) -> (21.5433, -51.6645)
  line L65 (21.5433, -51.6645) -> (21.8361, -52.3716)
  line L66 (21.8361, -52.3716) -> (18.2, -56.0077)
  line L67 (18.2, -56.0077) -> (18.2, -60.2)
  arc A5 (9.8, -60.2) -> (18.2, -60.2) centre (14, -60.2) ccw
  line L68 (9.8, -60.2) -> (9.8, -56.0077)
  line L69 (9.8, -56.0077) -> (6.1639, -52.3716)
  line L70 (6.1639, -52.3716) -> (6.4567, -51.6645)
  line L71 (6.4567, -51.6645) -> (8.2145, -51.6645)
  line L72 (8.2145, -51.6645) -> (11.75, -55.2)
  line L73 (11.75, -55.2) -> (11.75, -60.2)
  line L74 (21.8361, 68.0284) -> (22.0433, 68.2355)
  line L75 (6.1639, 68.0284) -> (5.9567, 68.2355)
  line L76 (88.6639, 68.0284) -> (88.4567, 68.2355)
  line L77 (104.3361, 68.0284) -> (104.5433, 68.2355)
  constraint coincident L14.end L15.start
  constraint midpoint L13 L74.end
  constraint coincident L18.end L19.start
  constraint midpoint L20 L75.end
  constraint coincident L5.end L6.start
  constraint midpoint L7 L76.end
  constraint coincident L1.end L2.start
  constraint midpoint L0 L77.end
extrude "Extrude7" add sketch "Fill In After Chamfer" along normal blind 5 contours L0 L1 L77 | L6 L7 L76 | L19 L20 L75 | L13 L14 L74 bodies 3 in component "End Frame A"
sketch "Sketch1" plane through (0, 7, 0) normal (0, 1, 0) x (-1, 0, 0) in component "Standoff for End Frame"
  line L0 (-26.9133, 50.2) -> (-55.25, 8.8457)
  line L1 (-55.25, 8.8457) -> (-83.5867, 50.2)
  line L2 (-83.5867, 50.2) -> (-26.9133, 50.2)
  line L3 (-61.3112, 0) -> (-95.709, -50.2)
  line L4 (-95.709, -50.2) -> (-98.2, -50.2)
  line L5 (-98.2, -50.2) -> (-98.2, 50.2)
  line L6 (-98.2, 50.2) -> (-95.709, 50.2)
  line L7 (-95.709, 50.2) -> (-61.3112, 0)
  line L8 (-14.791, -50.2) -> (-49.1888, 0)
  line L9 (-49.1888, 0) -> (-14.791, 50.2)
  line L10 (-14.791, 50.2) -> (-12.3, 50.2)
  line L11 (-12.3, 50.2) -> (-12.3, -50.2)
  line L12 (-12.3, -50.2) -> (-14.791, -50.2)
  line L13 (-26.9133, -50.2) -> (-83.5867, -50.2)
  line L14 (-83.5867, -50.2) -> (-55.25, -8.8457)
  line L15 (-55.25, -8.8457) -> (-26.9133, -50.2)
  circle A0 centre (-14, -60.2) radius 1.5
  circle A1 centre (-14, 60.2) radius 1.5
  circle A2 centre (-96.5, -60.2) radius 1.5
  circle A3 centre (-96.5, 60.2) radius 1.5
  line L16 (-104.0433, 68.7355) -> (-105.0433, 67.7355)
  line L17 (-105.0433, 67.7355) -> (-105.0433, 60.8567)
  line L18 (-105.0433, 60.8567) -> (-108.2, 57.7)
  line L19 (-108.2, 57.7) -> (-108.2, -57.7)
  line L20 (-108.2, -57.7) -> (-100.7, -65.2)
  line L21 (-100.7, -65.2) -> (-92.3, -65.2)
  line L22 (-92.3, -65.2) -> (-87.3, -60.2)
  line L23 (-87.3, -60.2) -> (-23.2, -60.2)
  line L24 (-23.2, -60.2) -> (-18.2, -65.2)
  line L25 (-18.2, -65.2) -> (-9.8, -65.2)
  line L26 (-9.8, -65.2) -> (-2.3, -57.7)
  line L27 (-2.3, -57.7) -> (-2.3, 57.7)
  line L28 (-2.3, 57.7) -> (-5.4567, 60.8567)
  line L29 (-5.4567, 60.8567) -> (-5.4567, 67.7355)
  line L30 (-5.4567, 67.7355) -> (-6.4567, 68.7355)
  line L31 (-6.4567, 68.7355) -> (-8.2145, 68.7355)
  line L32 (-8.2145, 68.7355) -> (-11.75, 65.2)
  line L33 (-11.75, 65.2) -> (-16.25, 65.2)
  line L34 (-16.25, 65.2) -> (-19.7855, 68.7355)
  line L35 (-19.7855, 68.7355) -> (-21.5433, 68.7355)
  line L36 (-21.5433, 68.7355) -> (-22.5433, 67.7355)
  line L37 (-22.5433, 67.7355) -> (-22.5433, 60.8567)
  line L38 (-22.5433, 60.8567) -> (-23.2, 60.2)
  line L39 (-23.2, 60.2) -> (-87.3, 60.2)
  line L40 (-87.3, 60.2) -> (-87.9567, 60.8567)
  line L41 (-87.9567, 60.8567) -> (-87.9567, 67.7355)
  line L42 (-87.9567, 67.7355) -> (-88.9567, 68.7355)
  line L43 (-88.9567, 68.7355) -> (-90.7145, 68.7355)
  line L44 (-90.7145, 68.7355) -> (-94.25, 65.2)
  line L45 (-94.25, 65.2) -> (-98.75, 65.2)
  line L46 (-98.75, 65.2) -> (-102.2855, 68.7355)
  line L47 (-102.2855, 68.7355) -> (-104.0433, 68.7355)
  circle A4 centre (-14, 60.2) radius 4.25
  circle A5 centre (-14, 60.2) radius 1.5
  dimension "d107" = 8.5
  constraint concentric A1 A4
  constraint concentric A4 A5
  measures "d107" diameter of A4
extrude "Extrude1'''" add sketch "Sketch1" along normal blind 2 separate body contours A1 A5 | A4 makes body 4 in component "Standoff for End Frame"
extrude "Extrude2''" add sketch "Sketch1" against normal blind 1.45 contours A1 A5 bodies 4 in component "Standoff for End Frame"